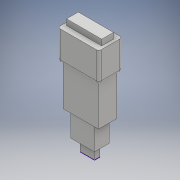
# Autodesk Inventor part: USB2Dynamixel-XD
Saved by Autodesk Inventor 2017 (Build 210142000, 142)
## iProperties
Created: 2017-10-29
Part Number: USB2Dynamixel-XD
Material: Ogólny
Document SubType Name: Modeling
Designer: Lenovo
Density: 1 g/cm^3
Appearance: Domyślna
Author: Lenovo
Autodesk Inventor part; units mm, degrees
ref_plane "YZ Plane" through (0, 0, 0) normal (1, 0, 0) x (0, 1, 0)
ref_plane "XZ Plane" through (0, 0, 0) normal (0, 1, 0) x (-1, 0, 0)
ref_plane "XY Plane" through (0, 0, 0) normal (0, 0, 1) x (1, 0, 0)
sketch "Szkic1" plane through (0, 0, 0) normal (0, 0, 1) x (1, 0, 0)
  line L0 (6, -2.25) -> (-6, -2.25)
  line L1 (-6, -2.25) -> (-6, 2.25)
  line L2 (-6, 2.25) -> (6, 2.25)
  line L3 (6, 2.25) -> (6, -2.25)
  line L4 (6, -2.25) -> (-6, 2.25) construction
  line L5 (-6, -2.25) -> (6, 2.25) construction
  line L6 (6, -2.25) -> (-6, -2.25)
  line L7 (-6, -2.25) -> (-6, 2.25)
  line L8 (-6, 2.25) -> (6, 2.25)
  line L9 (6, 2.25) -> (6, -2.25)
  line L10 (6, -2.25) -> (-6, 2.25) construction
  line L11 (-6, -2.25) -> (6, 2.25) construction
  point P0 (0, 0)
  dimension "d0" = 12
  dimension "d1" = 4.5
  constraints: 24 end point, 4 midpoint, 4 parallel, 2 horizontal, 2 perpendicular
  measures "d0" distance between parallel lines of L3 L1
  measures "d1" distance between parallel lines of L0 L2
extrude "Wyciągnięcie proste1" add sketch "Szkic1" against normal blind 10
sketch "Szkic2" plane through (0, 0, -10) normal (0, 0, -1) x (-1, 0, 0)
  line L0 (6, 2.25) -> (-6, 2.25) projected
  line L1 (6, -2.25) -> (-6, -2.25)
  line L2 (-6, -2.25) -> (-6, 2.25)
  line L3 (-6, 2.25) -> (6, 2.25)
  line L4 (6, 2.25) -> (6, -2.25)
  line L5 (6, -2.25) -> (-6, 2.25) construction
  line L6 (-6, -2.25) -> (6, 2.25) construction
  point P0 (0, 0)
  constraints: 12 end point, 2 midpoint, 2 parallel, 1 horizontal, 1 perpendicular
sketch "Szkic3" plane through (0, 0, 0) normal (0, 0, 1) x (1, 0, 0)
  line L0 (10, -6.25) -> (-10, -6.25)
  line L1 (-10, -6.25) -> (-10, 6.25)
  line L2 (-10, 6.25) -> (10, 6.25)
  line L3 (10, 6.25) -> (10, -6.25)
  line L4 (10, -6.25) -> (-10, 6.25) construction
  line L5 (-10, -6.25) -> (10, 6.25) construction
  point P0 (0, 0)
  dimension "d4" = 20
  dimension "d5" = 12.5
  constraints: 12 end point, 2 midpoint, 2 parallel, 1 horizontal, 1 perpendicular
  measures "d4" distance between parallel lines of L3 L1
  measures "d5" distance between parallel lines of L0 L2
extrude "Wyciągnięcie proste2" add sketch "Szkic3" along normal blind 20
sketch "Szkic5" plane through (0, 0, 20) normal (0, 0, 1) x (1, 0, 0)
  line L0 (15, -7.75) -> (-15, -7.75)
  line L1 (-15, -7.75) -> (-15, 7.75)
  line L2 (-15, 7.75) -> (15, 7.75)
  line L3 (15, 7.75) -> (15, -7.75)
  line L4 (15, -7.75) -> (-15, 7.75) construction
  line L5 (-15, -7.75) -> (15, 7.75) construction
  point P0 (0, 0)
  dimension "d8" = 15.5
  dimension "d9" = 30
  constraints: 12 end point, 2 midpoint, 2 parallel, 1 horizontal, 1 perpendicular
  measures "d8" distance between parallel lines of L0 L2
  measures "d9" distance between parallel lines of L1 L3
extrude "Wyciągnięcie proste3" add sketch "Szkic5" along normal blind 35
sketch "Szkic6" plane through (0, 0, 55) normal (0, 0, 1) x (1, 0, 0)
  line L0 (17.5, -10) -> (-17.5, -10)
  line L1 (-17.5, -10) -> (-17.5, 10)
  line L2 (-17.5, 10) -> (17.5, 10)
  line L3 (17.5, 10) -> (17.5, -10)
  line L4 (17.5, -10) -> (-17.5, 10) construction
  line L5 (-17.5, -10) -> (17.5, 10) construction
  point P0 (0, 0)
  dimension "d12" = 20
  dimension "d13" = 35
  constraints: 12 end point, 2 midpoint, 2 parallel, 1 horizontal, 1 perpendicular
  measures "d12" distance between parallel lines of L0 L2
  measures "d13" distance between parallel lines of L3 L1
extrude "Wyciągnięcie proste4" add sketch "Szkic6" along normal blind 25
sketch "Szkic7" plane through (0, 0, 80) normal (0, 0, 1) x (1, 0, 0)
  line L0 (15, -5) -> (-15, -5)
  line L1 (-15, -5) -> (-15, 5)
  line L2 (-15, 5) -> (15, 5)
  line L3 (15, 5) -> (15, -5)
  line L4 (15, -5) -> (-15, 5) construction
  line L5 (-15, -5) -> (15, 5) construction
  point P0 (0, 0)
  dimension "d16" = 10
  dimension "d17" = 30
  constraints: 12 end point, 2 midpoint, 2 parallel, 1 horizontal, 1 perpendicular
  measures "d16" distance between parallel lines of L0 L2
  measures "d17" distance between parallel lines of L3 L1
extrude "Wyciągnięcie proste5" add sketch "Szkic7" along normal blind 5
fillet "Zaokrąglenie1" radius 2 4 edges at (0, 10, 55) (-17.5, 0, 55) (17.5, 0, 55) (0, -10, 55)
fillet "Zaokrąglenie2" radius 2 8 edges at (16.9142, 9.4142, 55.5858) (17.5, 10, 68.5) (-16.9142, 9.4142, 55.5858) (-17.5, 10, 68.5) (16.9142, -9.4142, 55.5858) (17.5, -10, 68.5) (-16.9142, -9.4142, 55.5858) (-17.5, -10, 68.5)
